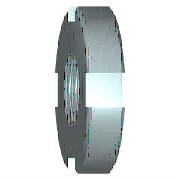
# Autodesk Inventor part: 螺母 GB 810 M64 x 2
Saved by Autodesk Inventor 2020 (Build 240168000, 168)
## iProperties
Created: 2019-01-21
Part Number: 螺母 GB 810 M64 x 2
Material: 钢，软
Description: 小圆螺母
Document SubType Name: Modeling
Standard: GB/T 810-1988
Designer: dell
Standard Revision: 1988
Standards Organization: GB
Language: zh-CN
Size Designation: M64x2
Categories: <MemberInstance><Categories><Category DisplayName="轴用零件" InternalName="7f7aeb1f-a693-4053-b835-cee3144e0d98" Mnemonic="SHFT"><Category DisplayName="圆螺母" InternalName="45a26349-4277-4297-8fe1-8d44e638a430" Mnemonic="NUTLCKELM"><CategoryParameter DisplayName="螺纹精度" InternalName="15b8a067-5188-4c64-a8c2-28b92b4a7cf6" Mnemonic="lnthrclss"/><CategoryParameter DisplayName="高度" InternalName="195ce0b8-bf58-4175-ab26-fbba4c9bf976" Mnemonic="lnheig"/><CategoryParameter DisplayName="接触区域直径" InternalName="2655266a-9fa5-4dcd-a57e-fd5caf012750" Mnemonic="conarea"/><CategoryParameter DisplayName="沟槽宽度" InternalName="8d288d8e-01ae-46e0-926b-ffde0badb65d" Mnemonic="grvwdth"/><CategoryParameter DisplayName="螺纹规格" InternalName="a9eb60e9-f1b0-4f14-b485-08820e33cf8c" Mnemonic="lnthrdesign"/><CategoryParameter DisplayName="轴直径" InternalName="c42cf996-bc5f-4e13-85af-dd5a70a2b8ac" Mnemonic="shaftdia"/><CategoryParameter DisplayName="螺纹系列规格" InternalName="d5956993-4017-4dc0-865f-74a86df05bb5" Mnemonic="lnthrserdsgn"/><CategoryParameter DisplayName="外径" InternalName="e074d5ef-539a-4177-b60b-1bcff90575aa" Mnemonic="outdia"/></Category></Category><Category DisplayName="数据类型" InternalName="23b78d0f-2648-40c6-8793-ca6db495c9e8" Mnemonic="DATATYPE"><CategoryParameter DisplayName="显示名" InternalName="05415f3d-3907-474b-a020-eb9d644f4cf3" Mnemonic="DISPLAYNAME"/><CategoryParameter DisplayName="标准" InternalName="0c0a119c-1e12-4c84-803f-101930972f5e" Mnemonic="STANDARD"/><CategoryParameter DisplayName="描述" InternalName="13903e3d-64b1-4950-80da-f627842ea37f" Mnemonic="DESCRIPTION"/><CategoryParameter DisplayName="规格" InternalName="2675968c-4ce5-49e0-a4f5-552d29089031" Mnemonic="DESIGNATION"/><CategoryParameter DisplayName="默认列" InternalName="2af9ec52-faaa-4026-b378-f9fa4afca842" Mnemonic="DEFAULTROW"/><CategoryParameter DisplayName="文件夹名称" InternalName="3f06958e-8713-4116-9be7-ed6184ecc97b" Mnemonic="FOLDERNAME"/><CategoryParameter DisplayName="版本指南" InternalName="45a75005-10b1-4dfc-8d6d-dfe629f0b93c" Mnemonic="REVISIONGUID"/><CategoryParameter DisplayName="文件名" InternalName="8b46a4cc-9585-4fed-90c3-899f57e09a73" Mnemonic="FILENAME"/><CategoryParameter DisplayName="标准组织" InternalName="8f5914e1-4693-403f-8ab5-d37768198c9d" Mnemonic="STDSORG"/><CategoryParameter DisplayName="系列版本" InternalName="914462f6-6e19-4b14-ba84-155b9680b1d0" Mnemonic="FAMILYREVISION"/><CategoryParameter DisplayName="标准版本" InternalName="91d5a463-65c2-4fde-b823-3b7fea5e8e17" Mnemonic="STANDARDREVISION"/><CategoryParameter DisplayName="成员版本" InternalName="a65d44b9-392f-4f4f-857b-e4b3d54996fe" Mnemonic="MEMBERREVISION"/><CategoryParameter DisplayName="剪裁格式" InternalName="bc51e27b-3422-4e78-93ef-cec197ddf230" Mnemonic="CLIPFORMAT"/><CategoryParameter DisplayName="制造商" InternalName="cd6c7a72-a28a-4e50-99a9-2c7f4e13e5ad" Mnemonic="MANUFACTURER"/><CategoryParameter DisplayName="内部名称" InternalName="cf1d0246-76d9-4b4a-8305-fa0409afb5c1" Mnemonic="INTERNALNAME"/><CategoryParameter DisplayName="是否公制" InternalName="e2385c5b-1ea4-4823-96a8-8de651266ec3" Mnemonic="ISMETRIC"/><Category DisplayName="零件" InternalName="c0e0b642-3bcb-4cc8-9e80-f96d35c4afa4" Mnemonic="PART"><CategoryParameter DisplayName="零件代号" InternalName="016b6077-bfbe-49bd-92c9-d8d59c39c941" Mnemonic="PARTNUMBER"/><CategoryParameter DisplayName="库存编号" InternalName="4dba7c1c-e26c-444e-836c-b08b433409a8" Mnemonic="STOCKNUMBER"/><CategoryParameter DisplayName="材料键" InternalName="5c9a8adb-dd2b-4535-b97f-0a94a95fe41f" Mnemonic="MATERIALKEY"/><CategoryParameter DisplayName="材料" InternalName="818a152a-d3c3-49ca-80ee-df7d91421b8e" Mnemonic="MATERIAL"/></Category></Category><Category DisplayName="先前版本映射" InternalName="cd87c42b-3e48-431e-b5c0-1cbeb14dfe77" Mnemonic="LEGACYMAP"><CategoryParameter DisplayName="唯一 DA 成员 ID" InternalName="0918ad47-427f-4fed-ae26-24c81c58f590" Mnemonic="DACOOKIE"/><CategoryParameter DisplayName="合并11 ID" InternalName="0ee8fb18-e2ed-4f39-96f6-1f4b5f50aa71" Mnemonic="MERGE11"/><CategoryParameter DisplayName="唯一 CC 成员 ID" InternalName="5193edd4-b2b0-4ab4-9d54-de900eee34e0" Mnemonic="CCCOOKIE"/><CategoryParameter DisplayName="分割 ID" InternalName="72b5c83c-be7f-45c4-ae51-9160ea6deb26" Mnemonic="SPLIT"/><CategoryParameter DisplayName="成员 ID" InternalName="8e5e0294-fc51-4c8f-b3d7-003dc5ed94f6" Mnemonic="MEMBERID"/><CategoryParameter DisplayName="目录名" InternalName="d99d1e27-aa94-4de2-af4c-c348882a6f4f" Mnemonic="CATALOGNAME"/><CategoryParameter DisplayName="系列编号" InternalName="e705e1f4-09cb-413e-91f9-551b4188271e" Mnemonic="FAMILYNUMBER"/></Category></Categories><FamilyTemplate Id="no0055"><FamilyTemplateParameters><FamilyTemplateParameter ObjectType="kUserParameterObject" ValueType="xs:double" Id="1" ObjectReferenceKey="GUL"/><FamilyTemplateParameter ObjectType="kUserParameterObject" ValueType="xs:double" Id="2" ObjectReferenceKey="KOH"/><FamilyTemplateParameter ObjectType="kUserParameterObject" ValueType="xs:double" Id="3" ObjectReferenceKey="TPU"/><FamilyTemplateParameter ObjectType="kUserParameterObject" ValueType="xs:double" Id="4" ObjectReferenceKey="PHH"/><FamilyTemplateParameter ObjectType="kUserParameterObject" ValueType="xs:double" Id="5" ObjectReferenceKey="SNT"/><FamilyTemplateParameter ObjectType="kUserParameterObject" ValueType="xs:double" Id="6" ObjectReferenceKey="NND"/><FamilyTemplateParameter ObjectType="kUserParameterObject" ValueType="xs:double" Id="7" ObjectReferenceKey="THREADDIA"/><FamilyTemplateParameter ObjectType="kUserParameterObject" ValueType="xs:double" Id="8" ObjectReferenceKey="SNB"/><FamilyTemplateParameter ObjectType="kUserParameterObject" ValueType="xs:double" Id="9" ObjectReferenceKey="TOA"/><FamilyTemplateParameter ObjectType="kUserParameterObject" ValueType="xs:double" Id="10" ObjectReferenceKey="FAWI"/><FamilyTemplateParameter ObjectType="kUserParameterObject" ValueType="xs:double" Id="11" ObjectReferenceKey="PTC"/><FamilyTemplateParameter ObjectType="kUserParameterObject" ValueType="xs:double" Id="12" ObjectReferenceKey="FAWI1"/><FamilyTemplateParameter ObjectType="kUserParameterObject" ValueType="xs:double" Id="13" ObjectReferenceKey="NAZ"/><FamilyTemplateParameter ObjectType="kUserParameterObject" ValueType="xs:double" Id="14" ObjectReferenceKey="LADI"/><FamilyTemplateParameter ObjectType="kUserParameterObject" ValueType="xs:double" Id="15" ObjectReferenceKey="GAL"/><FamilyTemplateParameter ObjectType="kUserParameterObject" ValueType="xs:double" Id="16" ObjectReferenceKey="SD2"/><FamilyTemplateParameter ObjectType="kUserParameterObject" ValueType="xs:double" Id="17" ObjectReferenceKey="GD1"/><FamilyTemplateParameter ObjectType="kPropertyObject" ValueType="xs:string" Id="100" ObjectReferenceKey="{32853F0F-3444-11d1-9E93-0060B03C1CA6}" SubObjectId="52"/><FamilyTemplateParameter ObjectType="kPropertyObject" ValueType="xs:string" Id="105" ObjectReferenceKey="{32853F0F-3444-11d1-9E93-0060B03C1CA6}" SubObjectId="5"/><FamilyTemplateParameter ObjectType="kPartComponentDefinitionObject" ValueType="xs:string" Id="110" SubObjectId="Material"/><FamilyTemplateParameter ObjectType="kThreadFeatureObject" ValueType="xs:structure" Id="300" ObjectReferenceKey="1002000010000000a4010000000000008000000000000000" SubObjectId="ThreadInfo"><FamilyTemplateParameter ObjectType="" ValueType="xs:string" Id="301" SubObjectId="ThreadDesignation"/><FamilyTemplateParameter ObjectType="" ValueType="xs:string" Id="302" SubObjectId="ThreadType"/><FamilyTemplateParameter ObjectType="" ValueType="xs:string" Id="303" SubObjectId="ThreadClass"/></FamilyTemplateParameter></FamilyTemplateParameters></FamilyTemplate><CategoryParameterMap><ParamToTemplateMap><ParamToTemplate CategoryParameter="//CategoryParameter[@InternalName='05415f3d-3907-474b-a020-eb9d644f4cf3']" ConstantValue="Nut GB/T 810-1988"/><ParamToTemplate CategoryParameter="//CategoryParameter[@InternalName='cf1d0246-76d9-4b4a-8305-fa0409afb5c1']" ConstantValue="a29d8a12-2b1e-4dce-bb6b-429f32aef0c0"/><ParamToTemplate CategoryParameter="//CategoryParameter[@InternalName='3f06958e-8713-4116-9be7-ed6184ecc97b']" ConstantValue="GB 810-88"/><ParamToTemplate CategoryParameter="//CategoryParameter[@InternalName='914462f6-6e19-4b14-ba84-155b9680b1d0']" ConstantValue="10"/><ParamToTemplate CategoryParameter="//CategoryParameter[@InternalName='bc51e27b-3422-4e78-93ef-cec197ddf230']" ConstantValue="CF_INVENTOR.STDPARTS"/><ParamToTemplate CategoryParameter="//CategoryParameter[@InternalName='e2385c5b-1ea4-4823-96a8-8de651266ec3']" ConstantValue="true"/><ParamToTemplate CategoryParameter="//CategoryParameter[@InternalName='13903e3d-64b1-4950-80da-f627842ea37f']" ConstantValue="Small round nuts"/><ParamToTemplate CategoryParameter="//CategoryParameter[@InternalName='8f5914e1-4693-403f-8ab5-d37768198c9d']" ConstantValue="GB"/><ParamToTemplate CategoryParameter="//CategoryParameter[@InternalName='0c0a119c-1e12-4c84-803f-101930972f5e']" ConstantValue="GB/T 810-1988"/><ParamToTemplate CategoryParameter="//CategoryParameter[@InternalName='cd6c7a72-a28a-4e50-99a9-2c7f4e13e5ad']" TemplateParameter="104"/><ParamToTemplate CategoryParameter="//CategoryParameter[@InternalName='91d5a463-65c2-4fde-b823-3b7fea5e8e17']" ConstantValue="1988"/><ParamToTemplate CategoryParameter="//CategoryParameter[@InternalName='45a75005-10b1-4dfc-8d6d-dfe629f0b93c']" ConstantValue="f703b5f1-e361-41ee-afb1-a15af7af8962"/><ParamToTemplate CategoryParameter="//CategoryParameter[@InternalName='2af9ec52-faaa-4026-b378-f9fa4afca842']" ConstantValue="10"/><ParamToTemplate CategoryParameter="//CategoryParameter[@InternalName='d99d1e27-aa94-4de2-af4c-c348882a6f4f']" ConstantValue="GB"/><ParamToTemplate CategoryParameter="//CategoryParameter[@InternalName='e705e1f4-09cb-413e-91f9-551b4188271e']" ConstantValue="310"/><ParamToTemplate CategoryParameter="//CategoryParameter[@InternalName='8b46a4cc-9585-4fed-90c3-899f57e09a73']" ConstantValue="螺母 GB 810 M64 x 2"/><ParamToTemplate CategoryParameter="//CategoryParameter[@InternalName='a65d44b9-392f-4f4f-857b-e4b3d54996fe']" ConstantValue="d82450a8-d87f-41cc-b4a8-9b3be9f23583"/><ParamToTemplate CategoryParameter="//CategoryParameter[@InternalName='15b8a067-5188-4c64-a8c2-28b92b4a7cf6']" ConstantValue="6H"/><ParamToTemplate CategoryParameter="//CategoryParameter[@InternalName='8e5e0294-fc51-4c8f-b3d7-003dc5ed94f6']" ConstantValue="200"/><ParamToTemplate CategoryParameter="//CategoryParameter[@InternalName='2675968c-4ce5-49e0-a4f5-552d29089031']" TemplateParameter="100"/><ParamToTemplate CategoryParameter="//CategoryParameter[@InternalName='195ce0b8-bf58-4175-ab26-fbba4c9bf976']" TemplateParameter="2"/><ParamToTemplate CategoryParameter="//CategoryParameter[@InternalName='818a152a-d3c3-49ca-80ee-df7d91421b8e']" TemplateParameter="110"/><ParamToTemplate CategoryParameter="//CategoryParameter[@InternalName='c42cf996-bc5f-4e13-85af-dd5a70a2b8ac']" TemplateParameter="6"/><ParamToTemplate CategoryParameter="//CategoryParameter[@InternalName='016b6077-bfbe-49bd-92c9-d8d59c39c941']" TemplateParameter="105"/><ParamToTemplate CategoryParameter="//CategoryParameter[@InternalName='a9eb60e9-f1b0-4f14-b485-08820e33cf8c']" TemplateParameter="301"/></ParamToTemplateMap></CategoryParameterMap></MemberInstance>
Density: 7.85 g/cm^3
Appearance: 半抛光
IsCustomPart: 1
Author: dell
Autodesk Inventor part; units mm, degrees
ref_plane "YZ Plane" through (0, 0, 0) normal (1, 0, 0) x (0, 1, 0)
ref_plane "XZ Plane" through (0, 0, 0) normal (0, 1, 0) x (-1, 0, 0)
sketch "草图1" plane through (0, 0, 0) normal (0, 0, 1) x (1, 0, 0)
  line L0 (0, 0) -> (10, 0)
  line L1 (0, 0) -> (0, 42.5)
  line L2 (0, 42.5) -> (10, 42.5)
  line L3 (10, 42.5) -> (10, 0)
  line L4 (0, 51) -> (0, -8.5) projected
  line L5 (-2, 0) -> (12, 0) projected
  dimension "d1" = 85
  dimension "d2" = 10
  constraints: 8 end point, 3 perpendicular, 2 coincident, 2 point on line, 1 collinear, 1 horizontal, 1 vertical
  measures "d1" diameter of L2 L0
  measures "d2" distance between parallel lines of L3 L1
revolve "轴承体" add sketch "草图1" angle 360 about axis through (0, 0, 0) along (1, 0, 0)
sketch "草图2" plane through (0, 0, 0) normal (-1, 0, 0) x (0, 0, 1)
  circle A0 centre (0, 0) radius 42.5 projected
  point P0 (0, 0)
  constraints: 1 coincident
hole "螺纹" at (0, 0, 0) direction (1, 0, 0) diameter 61.835 end through all thread size "M64x2" class "6H" standard "GB Metric profile"
sketch "草图3" plane through (10, 0, 0) normal (1, 0, 0) x (0, 0, -1)
  circle A0 centre (0, 0) radius 42.5 projected
  line L0 (-4, 42.3113) -> (-4, 39)
  line L1 (-4, 39) -> (4, 39)
  line L2 (4, 39) -> (4, 42.3113)
  line L3 (0, -59.5) -> (0, 59.5) projected
  line L4 (-59.5, 0) -> (59.5, 0) projected
  dimension "d12" = 4
  dimension "d13" = 4
  dimension "d14" = 39
  constraints: 6 end point, 2 point on circle, 2 vertical, 1 horizontal alignment, 1 parallel, 1 perpendicular
  measures "d12" distance between parallel lines of L3 L0
  measures "d13" distance between parallel lines of L3 L2
  measures "d14" distance between parallel lines of L4 L1
extrude "沟槽1" cut sketch "草图3" against normal through all contours L2 L1 L3 A0 | L3 L1 L0 A0
pattern_circular "IDS_ARRAYGROOVE{1}" count 4 over 360 about axis through (-10, 0, 0) along (1, 0, 0) of "沟槽1"
chamfer "倒角1" distance 1 angle 45 4 edges at (0, 30.052, -30.052) (0, 30.052, 30.052) (0, -30.052, -30.052) (0, -30.052, 30.052) measured on face at (0, -20.4276, -32.5865)
chamfer "倒角2" distance 1 angle 45 4 edges at (10, 30.052, 30.052) (10, 30.052, -30.052) (10, -30.052, -30.052) (10, -30.052, 30.052) measured on face at (10, -20.4276, -32.5865)
chamfer "倒角3" distance 1.6 angle 30 1 edges at (10, 0, -30.9175) measured on face at (10, 20.075, -32.0252)
chamfer "倒角4" distance 1.6 angle 30 1 edges at (0, 0, -30.9175) measured on face at (0, -20.075, -32.0252)
ref_plane "Work Plane1" through (120.6234, 0, 0) normal (0, 1, 0) x (-1, 0, 0)
equation "\"d1\" = SD2"
equation "\"d2\" = KOH"
equation "\"d12\" = 0.5 * SNB"
equation "\"d13\" = 0.5 * SNB"
equation "\"d14\" = 0.5 * SD2 - SNT"
equation "\"d10\" = -0.5 * LADI + 0.5 * SD2"
equation "\"d11\" = FAWI"
equation "\"d41\" = -0.5 * LADI + 0.5 * SD2"
equation "\"d25\" = -0.5 * LADI + 0.5 * SD2"
equation "\"d27\" = FAWI"
equation "\"d42\" = -0.5 * LADI + 0.5 * SD2"
equation "\"d18\" = 0.025 * NND"
equation "\"d43\" = 0.025 * NND"
equation "\"d20\" = 0.025 * NND"
equation "\"d44\" = 0.025 * NND"
equation "\"NND\" = 64"
equation "\"KOH\" = 10"
equation "\"SD2\" = 85"
equation "\"SNB\" = 8"
equation "\"SNT\" = 3.5"
equation "\"LADI\" = 83"
equation "\"FAWI\" = 45deg"
equation "\"GUL\" = 0.61345 * PTC"
equation "\"PHH\" = 1"
equation "\"THREADDIA\" = 64"
equation "\"TOA\" = 30deg"
equation "\"PTC\" = 2"
equation "\"FAWI1\" = 60deg"
equation "\"GAL\" = 0.61345 * PTC"
equation "\"GD1\" = THREADDIA - 1.2269 * PTC"
body "Solid1"
